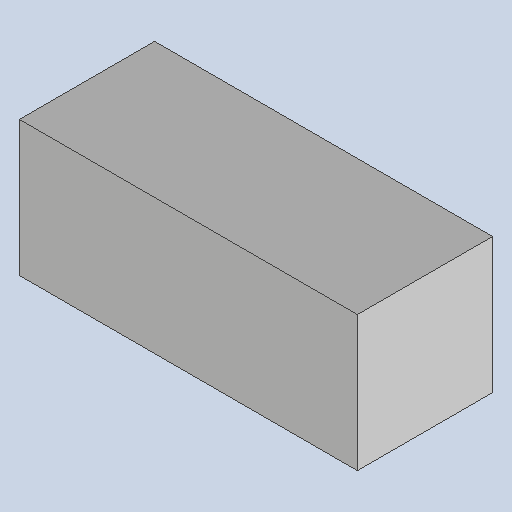
# Autodesk Inventor part: Bauteil8
Saved by Autodesk Inventor 2025 (Build 290162010, 162A)
## iProperties
Created: 2025-01-23
Part Number: Bauteil8
Material: OHNE_Pseudo-Teil
Document SubType Name: Modeling
Designer: Admin
Appearance: Vorgabe(2)
Author: Admin
Autodesk Inventor part; units mm, degrees
ref_plane "YZ Plane" through (0, 0, 0) normal (1, 0, 0) x (0, 1, 0)
ref_plane "XZ Plane" through (0, 0, 0) normal (0, 1, 0) x (-1, 0, 0)
ref_plane "XY Plane" through (0, 0, 0) normal (0, 0, 1) x (1, 0, 0)
sketch "Skizze1" plane through (0, 0, 0) normal (1, 0, 0) x (0, 1, 0)
  line L0 (0, 0) -> (-0.2, 0)
  line L1 (-0.2, 0) -> (-0.2, -0.2)
  line L2 (-0.2, -0.2) -> (0, -0.2)
  line L3 (0, -0.2) -> (0, 0)
  dimension "d3" = 0.2
  dimension "d4" = 0.2
  constraints: 8 end point, 2 parallel, 1 horizontal, 1 perpendicular
  measures "d3" distance of L2.end L1.end
  measures "d4" distance of L1.end L0.end
extrude "Extrusion1" add sketch "Skizze1" along normal blind 0.5
